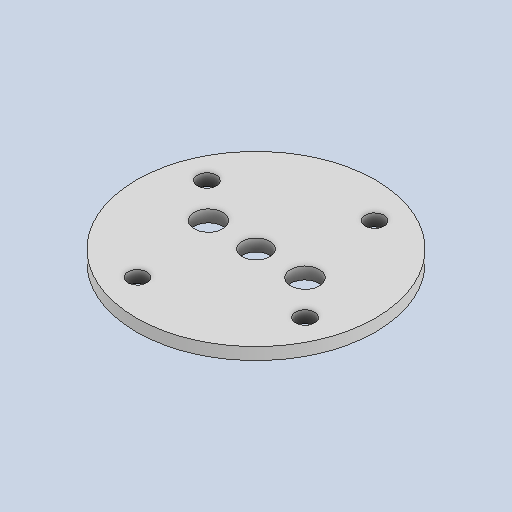
# Autodesk Inventor part: Prostavka
Saved by Autodesk Inventor 2023.2 (Build 272271030, 271C)
## iProperties
Created: 2023-12-24
Part Number: Prostavka
Material: Типовые
Document SubType Name: Modeling
Designer: Dell
Density: 1 g/cm^3
Appearance: По умолчанию
Mass: 14.1356 g
Surface Area: 82.8674 cm^2
Volume: 14.1356 cm^3
Author: Dell
Autodesk Inventor part; units mm, degrees
ref_plane "YZ Plane" through (0, 0, 0) normal (1, 0, 0) x (0, 1, 0)
ref_plane "XZ Plane" through (0, 0, 0) normal (0, 1, 0) x (-1, 0, 0)
ref_plane "XY Plane" through (0, 0, 0) normal (0, 0, 1) x (1, 0, 0)
sketch "Эскиз1" plane through (0, 0, 0) normal (0, 1, 0) x (-1, 0, 0)
  circle A0 centre (0, 0) radius 39.5
  circle A1 centre (0, 0) radius 4
  dimension "d0" = 79
  dimension "d3" = 8
  constraints: 2 centre point, 2 coincident
  measures "d0" diameter of A0
  measures "d3" diameter of A1
extrude "Выдавливание2" add sketch "Эскиз1" along normal blind 4
sketch "Эскиз3" plane through (0, 0, 0) normal (0, -1, 0) x (1, 0, 0)
  circle A0 centre (16.284, 0.1089) radius 4.75 projected
  circle A1 centre (-15.9974, -0.2901) radius 4.75 projected
  circle A2 centre (0, 0) radius 4.5
  dimension "d8" = 9
  constraints: 1 centre point, 1 coincident
  measures "d8" diameter of A2
extrude "Выдавливание3" cut sketch "Эскиз3" against normal blind 4
sketch "Эскиз4" plane through (0, 4, 0) normal (0, 1, 0) x (1, 0, 0)
  circle A0 centre (-27.7164, 11.4805) radius 4 construction
  circle A1 centre (-27.7164, 11.4805) radius 3.15
  point P0 (0, 0)
  dimension "d11" = 6.3
  constraints: 1 centre point, 1 coincident
  measures "d11" diameter of A1
extrude "Выдавливание4" cut sketch "Эскиз4" against normal blind 4
pattern_circular "Круговой массив1" count 4 over 360 about axis through (0, 0, 0) along (0, 1, 0) of "Выдавливание4"
